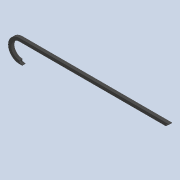
# Autodesk Inventor part: 0008-10-1026 wire chain Y
Saved by Autodesk Inventor 2020 (Build 240168000, 168)
## iProperties
Created: 2021-03-13
Part Number: 0008-10-1026 wire chain Y
Material: Generic
Document SubType Name: Modeling
Designer: Iulian Bors
Density: 1 g/cm^3
Appearance: Default
Description: Lant Portcablu
Mass: 33.8133 g
Surface Area: 340.239 cm^2
Volume: 33.8133 cm^3
Author: Iulian Bors
Subject: 1026
Autodesk Inventor part; units mm, degrees
ref_plane "YZ Plane" through (0, 0, 0) normal (1, 0, 0) x (0, 1, 0)
ref_plane "XZ Plane" through (0, 0, 0) normal (0, 1, 0) x (-1, 0, 0)
sketch "Sketch1" plane through (0, 0, 0) normal (0, 0, 1) x (1, 0, 0)
  line L0 (250, 69) -> (-250, 69)
  line L1 (-53.0332, 0) -> (53.0332, 0) construction
  arc A0 (-250, 69) -> (-250, 0) centre (-250, 34.5) ccw
  line L2 (-250, 0) -> (-240, 0)
  point P0 (0, 0)
  point P1 (0, 69)
  point P2 (0, 0)
  dimension "d0" = 500
  dimension "d1" = 69
  dimension "d25" = 10
  constraints: 6 end point, 2 horizontal, 2 midpoint, 2 point on circle, 2 tangent, 1 centre point, 1 coincident, 1 parallel, 1 point on line, 1 vertical alignment
  measures "d0" distance of L0.start L0.end
  measures "d1" distance between parallel lines of L1 L0
  measures "d25" distance of L2.start L2.end
ref_plane "Work Plane1" through (250, 69, 0) normal (-1, 0, 0) x (0, -1, 0)
sketch "Sketch2" plane through (250, 69, 0) normal (-1, 0, 0) x (0, -1, 0)
  line L0 (3.5, 3.5) -> (-3.5, 3.5)
  line L1 (-3.5, 3.5) -> (-3.5, -3.5)
  line L2 (-3.5, -3.5) -> (3.5, -3.5)
  line L3 (3.5, -3.5) -> (3.5, 3.5)
  line L4 (-5.5, 5.5) -> (5.5, 5.5)
  line L5 (5.5, 5.5) -> (5.5, -5.5)
  line L6 (5.5, -5.5) -> (-5.5, -5.5)
  line L7 (-5.5, -5.5) -> (-5.5, 5.5)
  point P0 (69, 0)
  point P1 (0, 3.5)
  point P2 (3.5, 0)
  point P3 (0, 0)
  point P4 (0, 0)
  point P5 (0, 0)
  dimension "d2" = 7
  dimension "d3" = 7
  dimension "d4" = 2
  constraints: 16 end point, 4 parallel, 2 midpoint, 2 perpendicular, 1 horizontal, 1 horizontal alignment, 1 vertical alignment, 3 other
  measures "d2" distance of L0.start L0.end
  measures "d3" distance of L0.end L1.end
  measures "d4" distance between parallel lines of L0 L4
sweep "Sweep1" add profiles "Sketch2" path "Sketch1"
sketch "Sketch3" plane through (250, 63.5, 5.5) normal (0, 0, 1) x (1, 0, 0)
  line L0 (0, 9) -> (-500, 9) projected
  line L1 (0, 9) -> (-10, 7.2367)
  line L2 (-10, 7.2367) -> (-10, 0)
  line L3 (0, 0) -> (-500, 0) projected
  line L4 (0, 0) -> (-500, 0) projected
  line L5 (0, 0) -> (0, 11) projected
  line L6 (-500, -67) -> (-490, -67) projected
  line L7 (-490, -67) -> (-500, -65.2367)
  line L8 (-500, -65.2367) -> (-500, -58)
  line L9 (-490, -58) -> (-490, -69) projected
  line L10 (-500, -58) -> (-490, -58) projected
  dimension "d29" = 100
  dimension "d30" = 10
  dimension "d33" = 100
  dimension "d34" = 10
  constraints: 8 end point, 2 point on line, 1 perpendicular
  measures "d29" angle of L2 L1
  measures "d30" distance between parallel lines of L5 L2
  measures "d33" angle of L7 L8
  measures "d34" distance between parallel lines of L8 L9
extrude "Extrusion1" cut sketch "Sketch3" against normal through all
body "Solid1"
